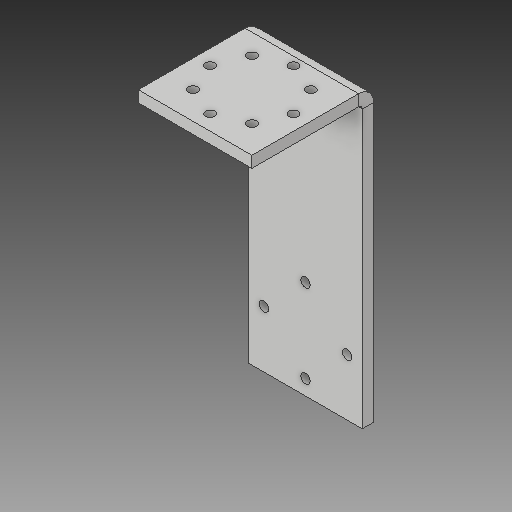
# Autodesk Inventor part: humerus
Saved by Autodesk Inventor 2018 (Build 220112000, 112)
## iProperties
Created: 2018-04-22
Part Number: humerus
Material: Generic
Document SubType Name: Sheet Metal
Designer: medrimonia
Density: 1 g/cm^3
Sheet Metal Rule: Default_mm
Appearance: Default
Vendor: Rhoban
Mass: 9.29873 g
Surface Area: 72.9359 cm^2
Volume: 9.29873 cm^3
Author: medrimonia
Autodesk Inventor part; units mm, degrees
ref_plane "YZ Plane" through (0, 0, 0) normal (1, 0, 0) x (0, 1, 0)
ref_plane "XZ Plane" through (0, 0, 0) normal (0, 1, 0) x (-1, 0, 0)
ref_plane "XY Plane" through (0, 0, 0) normal (0, 0, 1) x (1, 0, 0)
sketch "Sketch1" plane through (0, 0, 0) normal (0, 1, 0) x (-1, 0, 0)
  line L0 (-15, 30) -> (15, 30)
  line L1 (15, 30) -> (15, -75)
  line L2 (15, -75) -> (-15, -75)
  line L3 (-15, -75) -> (-15, 30)
  line L4 (-15, 0) -> (15, 0)
  line L5 (0, 30) -> (0, 0) construction
  line L6 (0, 15) -> (11, 15) construction
  line L7 (0, -75) -> (0, 0) construction
  line L8 (0, -60) -> (11, -60) construction
  point P0 (7.7782, 22.7782)
  point P1 (0, 26)
  point P2 (-7.7782, 22.7782)
  point P3 (-11, 15)
  point P4 (-7.7782, 7.2218)
  point P5 (0, 4)
  point P6 (7.7782, 7.2218)
  point P7 (0, -49)
  point P8 (-11, -60)
  point P9 (0, -71)
  dimension "d0" = 30
  dimension "d1" = 30
  dimension "d2" = 75
  dimension "d3" = 11
  dimension "d6" = 360
  dimension "d9" = 11
  dimension "d10" = 15
  dimension "d13" = 360
  constraints: 18 end point, 5 midpoint, 3 perpendicular, 3 point on line, 2 coincident, 2 horizontal, 2 parallel, 1 collinear, 1 vertical, 14 other
  measures "d0" distance between parallel lines of L0 L4
  measures "d1" distance of L0.start L0.end
  measures "d2" distance between parallel lines of L4 L2
  measures "d3" distance of L6.start L6.end
  measures "d9" distance of L8.start L8.end
  measures "d10" distance between parallel lines of L2 L8
extrude "Plate1" add sketch "Sketch1" along normal blind 3
hole "Hole1" at (-11, 0, 15) at (-7.7782, 0, 22.7782) at (0, 0, 26) at (7.7782, 0, 22.7782) at (11, 0, 15) at (7.7782, 0, 7.2218) at (0, 0, 4) at (-7.7782, 0, 7.2218) at (-11, 0, -60) at (0, 0, -49) at (11, 0, -60) at (0, 0, -71) direction (0, 1, 0) diameter 2.5 end through all
fold "Fold1" angle 90 bend radius 1 thickness 3 k factor 0.44 line from (15, 0, 0) to (-15, 0, 0) line at bend centre moving side (0, 0, -1) folds toward (0, -1, 0)
equation "\"d0\" = fix_length"
equation "\"d1\" = width"
equation "\"d2\" = humerus_length"
equation "\"d20\" = Thickness"
equation "\"d8\" = Thickness"
equation "\"d22\" = BendReliefWidth"
equation "\"d23\" = BendReliefDepth"
equation "\"d24\" = MinimumRemnant"
equation "\"d25\" = TransitionRadius"
equation "\"Thickness\" = thickness"
equation "\"BendRadius\" = Thickness"
equation "\"BendReliefWidth\" = Thickness"
equation "\"BendReliefDepth\" = 0.5 * Thickness"
equation "\"CornerReliefSize\" = 4 * Thickness"
equation "\"MinimumRemnant\" = 2 * Thickness"
equation "\"TransitionRadius\" = BendRadius"
equation "\"JacobiRadiusSize\" = BendRadius"
equation "\"GapSize\" = Thickness"
equation "\"fix_length\" = 30"
equation "\"width\" = 30"
equation "\"humerus_length\" = 75"
equation "\"thickness\" = 3"
body "Solid1"
